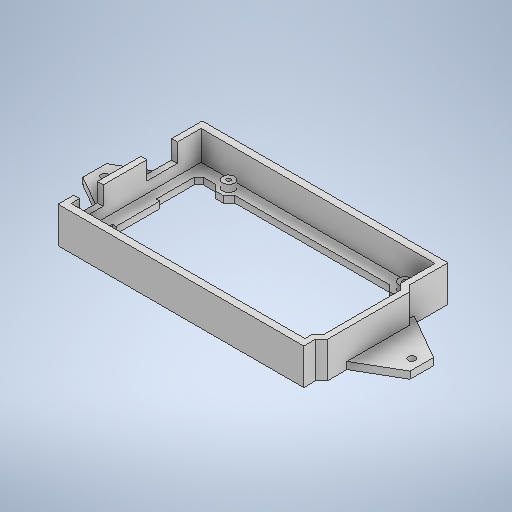
# Autodesk Inventor part: CaseArduinoMega
Saved by Autodesk Inventor 2025 (Build 290162000, 162)
## iProperties
Created: 2025-03-14
Part Number: CaseArduinoMega
Material: Genérico
Document SubType Name: Modeling
Designer: Ian
Density: 1 g/cm^3
Appearance: Padrão
Author: Ian
Autodesk Inventor part; units mm, degrees
ref_plane "YZ Plane" through (0, 0, 0) normal (1, 0, 0) x (0, 1, 0)
ref_plane "XZ Plane" through (0, 0, 0) normal (0, 1, 0) x (-1, 0, 0)
ref_plane "XY Plane" through (0, 0, 0) normal (0, 0, 1) x (1, 0, 0)
sketch "Esboço1" plane through (49, 0, -28.8005) normal (0, 1, 0) x (-1, 0, 0)
  line L0 (0, 16.5494) -> (0, 0)
  line L1 (0, 0) -> (0, 16.5494)
  line L2 (-2.54, 53.6742) -> (-2.54, 19.0894)
  line L3 (0, 16.5494) -> (-2.54, 19.0894)
  line L4 (-2.54, 19.0894) -> (-2.54, 53.6742)
  line L5 (-2.54, 53.6742) -> (0, 56.2142)
  line L6 (0, 56.2142) -> (0, 61.34)
  line L7 (104.54, 61.34) -> (104.54, 61.6011)
  line L8 (0, 61.34) -> (104.54, 61.34)
  line L9 (104.54, 61.34) -> (104.54, 0)
  line L10 (104.54, 0) -> (0, 0)
  line L11 (2.6222, 4.4772) -> (2.6222, 4.6028)
  line L12 (3.4259, 5.4351) -> (3.5514, 5.4395)
  circle A0 centre (11.8701, 6.54) radius 0.8973
  line L13 (8.9722, 52.7372) -> (8.9722, 52.8628)
  line L14 (9.7759, 53.6951) -> (9.9014, 53.6995)
  circle A1 centre (5.5202, 54.8) radius 0.8973
  line L15 (33.1022, 9.5572) -> (33.1022, 9.6828)
  line L16 (36.0001, 22.7395) -> (35.8746, 22.7351)
  circle A2 centre (35.9687, 21.84) radius 0.9
  line L17 (33.1022, 37.5628) -> (33.1022, 37.4372)
  line L18 (34.0314, 38.3995) -> (33.9059, 38.3951)
  circle A3 centre (36, 49.72) radius 0.8973
  line L19 (85.1722, 4.4772) -> (85.1722, 4.6028)
  line L20 (86.7372, 7.4351) -> (86.8627, 7.4395)
  circle A4 centre (86.8, 6.54) radius 0.9016
  circle A5 centre (88.07, 54.8) radius 0.8973
  dimension "d38" = 61.34
  dimension "d39" = 107.08
  dimension "d56" = 6.54
  dimension "d57" = 5.5202
  dimension "d58" = 6.54
  dimension "d60" = 21.84
  dimension "d61" = 38.5087
  dimension "d62" = 11.62
  dimension "d63" = 38.54
  dimension "d64" = 6.54
  dimension "d66" = 6.54
  dimension "d94" = 5.1258
  dimension "d95" = 16.5494
  dimension "d120" = 11.8701
  dimension "d121" = 16.47
  dimension "d122" = 17.74
  constraints: 42 end point, 4 centre point, 3 perpendicular, 2 collinear, 1 horizontal, 1 point on line, 1 vertical, 6 other
  measures "d38" distance between parallel lines of L10 L8
  measures "d39" distance between parallel lines of L9 L4
  measures "d56" distance from line of L8 A1.centre
  measures "d57" distance from line of L6 A1.centre
  measures "d58" distance from line of L10 A0.centre
  measures "d60" distance from line of L10 point (35.969, 21.84)
  measures "d61" distance from line of L2 point (35.969, 21.84)
  measures "d62" distance from line of L8 A3.centre
  measures "d63" distance from line of L2 A3.centre
  measures "d64" distance from line of L8 A5.centre
  measures "d66" distance from line of L10 point (86.8, 6.54)
  measures "d94" distance of L6.end L5.end
  measures "d95" distance of L0.end L0.start
  measures "d120" distance from line of L0 A0.centre
  measures "d121" distance from line of L9 A5.centre
  measures "d122" distance from line of L9 point (86.8, 6.54)
extrude "Extrusão1" add sketch "Esboço1" along normal blind 2.828
sketch "Esboço2" plane through (49, 2.828, -28.8005) normal (0, 1, 0) x (1, 0, 0)
  line L0 (-102.04, -58.34) -> (-102.04, -3)
  line L1 (0, 0) -> (-104.54, 0) projected
  line L2 (-104.54, -61.34) -> (0, -61.34) projected
  line L3 (-104.54, 0) -> (-104.54, -61.34) projected
  line L4 (-102.04, -3) -> (-2.5, -3)
  line L5 (-2.5, -58.34) -> (-102.04, -58.34)
  line L6 (-8.7044, -3) -> (1.4543, -3) construction
  line L7 (-2.5, -55.1787) -> (-2.5, -58.34)
  line L8 (2.54, -19.0894) -> (0, -16.5494) projected
  line L9 (2.54, -53.6742) -> (2.54, -19.0894) projected
  line L10 (0, -56.2142) -> (2.54, -53.6742) projected
  line L11 (0, -61.34) -> (0, -56.2142) projected
  line L12 (0, -16.5494) -> (0, 0) projected
  line L13 (0, 0) -> (0, -16.5494)
  line L14 (2.54, -19.0894) -> (2.54, -53.6742)
  line L15 (0, -56.2142) -> (0, -61.34)
  line L16 (-2.5, -55.1787) -> (0, -52.6787)
  line L17 (0, -20.0849) -> (-2.5, -17.5849)
  line L18 (-2.5, -17.5849) -> (-2.5, -3)
  line L19 (2.54, -19.0894) -> (0, -16.5494)
  line L20 (0, -20.0849) -> (0, -52.6787)
  point P0 (-49, -28.8005)
  point P1 (1.27, -54.9442)
  dimension "d3" = 3
  dimension "d4" = 3
  dimension "d6" = 2.5
  dimension "d15" = 2.5
  dimension "d96" = 2.5
  dimension "d97" = 2.5
  dimension "d98" = 2.5
  constraints: 26 end point, 4 parallel, 3 point on line, 2 collinear, 2 horizontal, 2 perpendicular, 2 vertical, 1 midpoint
  measures "d3" distance from line of L1 L0.end
  measures "d4" distance from line of L2 L0.start
  measures "d6" distance between parallel lines of L3 L0
  measures "d15" distance between parallel lines of L11 L7
  measures "d96" distance from line of point (1.27, -54.944) L16
  measures "d97" distance between parallel lines of L12 L18
  measures "d98" distance between parallel lines of L8 L17
extrude "Extrusão4" add sketch "Esboço2" along normal blind 12.5
sketch "Esboço5" plane through (-55.54, 0, -28.8005) normal (-1, 0, 0) x (0, 0, 1)
  line L0 (0, 0) -> (0, 15.328) projected
  line L1 (53.6742, 15.328) -> (19.0894, 15.328) projected
  line L2 (13.04, 15.328) -> (13.04, 7.478)
  line L3 (13.04, 7.478) -> (26.08, 7.478)
  line L4 (26.08, 7.478) -> (26.08, 15.328)
  line L5 (19.0894, 15.328) -> (26.08, 15.328)
  line L6 (55.1787, 15.328) -> (58.34, 15.328) projected
  line L7 (54.665, 15.328) -> (54.665, 7.478)
  line L8 (61.34, 0) -> (61.34, 15.328) projected
  line L9 (54.665, 7.478) -> (44.665, 7.478)
  line L10 (44.665, 7.478) -> (44.665, 15.328)
  line L11 (54.665, 15.328) -> (44.665, 15.328)
  line L12 (13.04, 15.328) -> (26.08, 15.328)
  line L13 (3, 15.328) -> (17.5849, 15.328) projected
  point P0 (28.8005, 0)
  point P1 (44.665, 11.403)
  point P2 (41.9718, 15.328)
  dimension "d45" = 13.04
  dimension "d46" = 13.04
  dimension "d47" = 7.85
  dimension "d49" = 7.85
  dimension "d50" = 6.675
  dimension "d51" = 10
  dimension "d52" = 18.585
  dimension "d53" = 61.34
  constraints: 18 end point, 4 point on line, 3 collinear, 3 perpendicular, 2 horizontal, 1 midpoint, 1 vertical
  measures "d45" distance between parallel lines of L0 L2
  measures "d46" distance of L2.end L3.end
  measures "d47" distance of L2.start L2.end
  measures "d49" distance of L7.start L7.end
  measures "d50" distance between parallel lines of L8 L7
  measures "d51" distance of L7.end L9.end
  measures "d52" distance from line of point (44.665, 11.403) L4
  measures "d53" distance between parallel lines of L8 L0
extrude "Extrusão5" cut sketch "Esboço5" against normal blind 12.5
sketch "Esboço7" plane through (-55.54, 0, -28.8005) normal (-1, 0, 0) x (0, 0, 1)
  line L0 (12.5489, 15.328) -> (31.9207, 15.328) projected
  line L1 (53.6742, 0) -> (19.0894, 0) projected
  line L2 (23.7839, 0) -> (33.7839, 0)
  line L3 (33.7839, 0) -> (33.7839, 3)
  line L4 (33.7839, 3) -> (23.7839, 3)
  line L5 (23.7839, 3) -> (23.7839, 0)
  point P0 (28.8005, 0)
  point P1 (39.5116, 15.328)
  point P2 (28.7839, 3)
  point P3 (28.7839, 0)
  point P4 (33.7839, 0)
  dimension "d68" = 10
  dimension "d69" = 3
  constraints: 8 end point, 2 midpoint, 2 parallel, 1 horizontal, 1 perpendicular, 1 point on line, 1 vertical alignment
  measures "d68" distance of L4.end L3.end
  measures "d69" distance of L3.end L2.end
extrude "Extrusão6" add sketch "Esboço7" along normal blind 17
sketch "Esboço10" plane through (51.54, 0, 24.8737) normal (1, 0, 0) x (0, 0, -1)
  line L0 (18.0042, 3) -> (28.0042, 3)
  line L1 (28.0042, 3) -> (28.0042, 0)
  line L2 (28.0042, 0) -> (18.0042, 0)
  line L3 (18.0042, 0) -> (18.0042, 3)
  line L4 (-7.6658, 15.328) -> (-2.54, 15.328) projected
  line L5 (-2.54, 15.328) -> (0, 15.328) projected
  line L6 (0, 15.328) -> (34.5848, 15.328) projected
  line L7 (34.5848, 15.328) -> (37.1248, 15.328) projected
  line L8 (37.1248, 15.328) -> (53.6742, 15.328) projected
  line L9 (-7.6658, 15.328) -> (53.6742, 15.328)
  line L10 (23.0042, 15.328) -> (23.0042, 6.8556)
  line L11 (-7.6658, 0) -> (-7.6658, 15.328) projected
  line L12 (0, 0) -> (34.5848, 0) projected
  point P0 (24.8737, 0)
  point P1 (23.0042, 3)
  dimension "d80" = 10
  dimension "d81" = 3
  dimension "d83" = 61.34
  dimension "d84" = 30.67
  dimension "d85" = 0
  dimension "d103" = 0
  constraints: 12 end point, 2 horizontal, 2 midpoint, 2 parallel, 2 perpendicular
  measures "d80" distance of L1.end L2.end
  measures "d81" distance of L0.end L1.end
  measures "d83" distance of L8.end L4.start
  measures "d84" distance between parallel lines of L11 L10
  measures "d85" distance from line of point (23.004, 3) L10
  measures "d103" distance between parallel lines of L12 L2
extrude "Extrusão9" add sketch "Esboço10" along normal blind 17
sketch "Esboço11" plane through (51.54, 3, 6.8695) normal (0, 1, 0) x (1, 0, 0)
  line L0 (17, 0) -> (17, 10) projected
  line L1 (-2.54, 19.1206) -> (-2.54, 35.67) projected
  line L2 (-2.54, 19.1206) -> (-2.54, 35.67) projected
  line L3 (0, 10) -> (17, 10) projected
  line L4 (17, 10) -> (-2.54, 21.2814)
  line L5 (0, -18.0042) -> (0, 16.5806) projected
  line L6 (17, 0) -> (0, -9.815)
  line L7 (0, 0) -> (17, 0) projected
  line L8 (0, 16.5806) -> (-2.54, 19.1206) projected
  line L9 (-2.54, 19.1206) -> (0, 16.5806)
  line L10 (-2.54, 21.2814) -> (-2.54, 19.1206)
  point P0 (-51.54, 6.8695)
  point P1 (-2.54, 21.2814)
  dimension "d99" = 30
  dimension "d100" = 30
  constraints: 8 end point, 2 collinear, 2 point on line
  measures "d99" angle of L3 L4
  measures "d100" angle of L6 L7
extrude "Extrusão11" add sketch "Esboço11" against normal up to surface (3 mm away) contours L6 L5 L7 | L3 L5 L8 L1 L4
sketch "Esboço12" plane through (-55.54, 3, 4.9834) normal (0, 1, 0) x (1, 0, 0)
  line L0 (0, 7.7039) -> (0, 20.7439) projected
  line L1 (-17, 10) -> (-17, 0) projected
  line L2 (-17, 0) -> (0, -9.815)
  line L3 (0, -20.8811) -> (0, -10.8811) projected
  line L4 (0, 10) -> (-17, 10) projected
  line L5 (-17, 10) -> (0, 19.815)
  line L6 (0, 0) -> (-17, 0) projected
  line L7 (0, 19.815) -> (0, 10)
  line L8 (0, 7.7039) -> (0, -10.8811) projected
  line L9 (-17, 10) -> (0, 10)
  line L10 (-17, 0) -> (0, 0)
  line L11 (0, -9.815) -> (0, 0)
  point P0 (55.54, 4.9834)
  dimension "d105" = 30
  dimension "d106" = 30
  constraints: 12 end point, 3 collinear, 2 point on line, 1 perpendicular
  measures "d105" angle of L4 L5
  measures "d106" angle of L6 L2
extrude "Extrusão12" add sketch "Esboço12" against normal up to surface (3 mm away) contours L4 L5 L0 | L8 L2 L6
sketch "Esboço13" plane through (-55.54, 3, 14.7983) normal (0, 1, 0) x (1, 0, 0)
  line L0 (0, -11.0661) -> (0, -1.0661) projected
  line L1 (-17, 9.815) -> (-17, 19.815) projected
  line L2 (0, 17.5189) -> (0, -1.0661) projected
  line L3 (0, 29.6299) -> (-17, 19.815) projected
  circle A0 centre (-12.75, 14.815) radius 1.5
  line L4 (124.08, 17.9289) -> (124.08, 7.9289) projected
  line L5 (107.08, -1.8861) -> (107.08, 24.5095) projected
  circle A1 centre (119.83, 12.9289) radius 1.5
  point P0 (55.54, 14.7983)
  dimension "d109" = 3
  dimension "d110" = 3
  constraints: 2 centre point
  measures "d109" diameter of A0
  measures "d110" diameter of A1
extrude "Extrusão13" cut sketch "Esboço13" against normal blind 10
sketch "Esboço14" plane through (49, 2.828, -28.8005) normal (0, 1, 0) x (1, 0, 0)
  circle A0 centre (-86.8, -6.54) radius 0.9016 projected
  circle A1 centre (-86.8, -6.54) radius 2.5
  circle A2 centre (-11.8701, -6.54) radius 0.8973 projected
  circle A3 centre (-11.8701, -6.54) radius 2.5
  circle A4 centre (-35.9687, -21.84) radius 0.9 projected
  circle A5 centre (-35.9687, -21.84) radius 2.5
  circle A6 centre (-88.07, -54.8) radius 0.8973 projected
  circle A7 centre (-88.07, -54.8) radius 2.5
  circle A8 centre (-36, -49.72) radius 0.8973 projected
  circle A9 centre (-36, -49.72) radius 2.5
  circle A10 centre (-5.5202, -54.8) radius 0.8973 projected
  circle A11 centre (-5.5202, -54.8) radius 2.5
  circle A12 centre (-36, -49.72) radius 0.8973 projected
  point P0 (-49, -28.8005)
  dimension "d113" = 5
  constraints: 6 centre point, 6 coincident, 3 equal radius
  measures "d113" diameter of A1
extrude "Extrusão14" add sketch "Esboço14" along normal blind 3
sketch "Esboço16" plane through (-39.07, 5.828, 25.9995) normal (0, 1, 0) x (1, 0, 0)
  line L0 (-13.97, 0.135) -> (-16.47, 0.135) projected
  line L1 (-16.47, 10.135) -> (-13.97, 10.135) projected
  line L2 (-13.97, 28.72) -> (-16.47, 28.72) projected
  line L3 (-16.47, 41.76) -> (-13.97, 41.76) projected
  line L4 (-9.97, 28.72) -> (-9.97, 44.8)
  line L5 (-8.47, 10.1069) -> (-8.47, 28.72)
  line L6 (85.57, -3.54) -> (-13.97, -3.54) projected
  line L7 (-13.97, 10.135) -> (-13.97, 0.135) projected
  line L8 (-7.9657, 46.8) -> (-2.8747, 46.8)
  line L9 (-0.3747, 44.3) -> (2.9148, 44.3)
  line L10 (5.4148, 46.8) -> (71.0558, 46.8)
  line L11 (88.07, 54.8) -> (-16.47, 54.8) projected
  line L12 (-16.47, -6.54) -> (88.07, -6.54) projected
  line L13 (90.61, 1.1258) -> (90.61, 35.7106) projected
  line L14 (-16.47, 28.72) -> (-16.47, 41.76) projected
  line L15 (-16.47, 28.72) -> (-16.47, 10.135) projected
  line L16 (-13.97, 51.8) -> (85.57, 51.8) projected
  circle A0 centre (1.2701, 48.26) radius 0.9016 projected
  circle A1 centre (0, 0) radius 0.8973 projected
  line L17 (-2.0287, 3.96) -> (2.0287, 3.96)
  line L18 (4.5287, 1.46) -> (77.3225, 1.46)
  line L19 (77.3225, 1.46) -> (78.4035, 1.46)
  line L20 (85.57, 51.8) -> (85.57, 37.2151) projected
  line L21 (85.57, 37.2151) -> (88.07, 34.7151) projected
  line L22 (88.07, 34.7151) -> (88.07, 2.1213) projected
  line L23 (80.07, 43.0238) -> (80.07, 35.7151)
  line L24 (80.07, 35.7151) -> (84.11, 31.3245)
  line L25 (84.11, 31.3245) -> (84.11, 6.8739)
  line L26 (80.07, 44.3) -> (80.07, 43.0238)
  line L27 (84.11, 3.96) -> (84.11, 6.8739)
  line L28 (73.5558, 44.3) -> (80.07, 44.3)
  circle A2 centre (76.2, 48.26) radius 0.8973 projected
  line L29 (73.7, 1.46) -> (77.7, 1.46) construction
  line L30 (78.4035, 1.46) -> (80.9035, 3.96)
  line L31 (78.4035, 1.46) -> (81.9391, 1.46) construction
  line L32 (80.9035, 3.96) -> (84.11, 3.96)
  line L33 (-16.47, 0.135) -> (-16.47, 10.135) projected
  line L34 (-9.97, 10.1069) -> (-8.47, 10.1069)
  line L35 (-9.97, 28.72) -> (-8.47, 28.72)
  line L36 (-7.9657, 46.8) -> (-7.97, 46.8)
  line L37 (-9.97, 44.8) -> (-7.97, 46.8)
  line L38 (-9.97, 44.8) -> (-7.1415, 44.8) construction
  line L39 (88.07, 38.2506) -> (88.07, 54.8) projected
  line L40 (71.0558, 46.8) -> (74.7636, 46.8) construction
  line L41 (71.0558, 46.8) -> (73.5558, 44.3)
  line L42 (71.0558, 46.8) -> (75.3342, 46.8) construction
  line L43 (-2.8747, 46.8) -> (-0.3747, 44.3)
  line L44 (2.9148, 44.3) -> (5.4148, 46.8)
  line L45 (-4.5287, 1.46) -> (-7.97, 1.46)
  line L46 (-4.5287, 1.46) -> (-2.0287, 3.96)
  line L47 (2.0287, 3.96) -> (4.5287, 1.46)
  line L48 (-9.97, 10.1069) -> (-9.97, 3.46)
  line L49 (-7.97, 1.46) -> (-9.97, 3.46)
  point P0 (39.07, 25.9995)
  point P1 (-9.97, 41.76)
  point P2 (1.2701, 44.3)
  point P3 (0, 3.96)
  point P4 (-15.22, 0.135)
  point P5 (-16.47, 35.24)
  point P6 (72.07, 46.8)
  point P7 (71.5558, 46.8)
  dimension "d131" = 8
  dimension "d157" = 6.5
  dimension "d158" = 8
  dimension "d162" = 2
  dimension "d165" = 8
  dimension "d166" = 6.5
  dimension "d167" = 8
  dimension "d170" = 2.5
  dimension "d172" = 2.5
  dimension "d173" = 2.5
  dimension "d174" = 2.5
  dimension "d175" = 2.5
  dimension "d176" = 2.5
  dimension "d177" = 2.5
  dimension "d180" = 8
  dimension "d181" = 2.5
  dimension "d182" = 2.5
  dimension "d183" = 2.5
  dimension "d184" = 2
  dimension "d185" = 2
  dimension "d186" = 2
  constraints: 66 end point, 11 horizontal, 6 parallel, 6 point on line, 4 midpoint, 4 perpendicular, 2 collinear, 2 equal length, 2 vertical, 2 vertical alignment
  measures "d131" distance between parallel lines of L11 L10
  measures "d157" distance from line of L4 point (-16.47, 35.24)
  measures "d158" distance between parallel lines of L15 L5
  measures "d162" horizontal distance of L4.end L36.end
  measures "d165" distance between parallel lines of L12 L18
  measures "d166" distance between parallel lines of L13 L25
  measures "d167" distance between parallel lines of L39 L23
  measures "d170" distance between parallel lines of L10 L28
  measures "d172" distance between parallel lines of L9 L8
  measures "d173" horizontal distance of L8.end L9.start
  measures "d174" horizontal distance of L9.end L10.start
  measures "d175" distance between parallel lines of L18 L17
  measures "d176" horizontal distance of L45.start L17.start
  measures "d177" horizontal distance of L17.end L18.start
  measures "d180" distance from line of point (72.07, 46.8) L23
  measures "d181" horizontal distance of L19.end L30.end
  measures "d182" distance between parallel lines of L32 L19
  measures "d183" horizontal distance of L10.end L28.start
  measures "d184" horizontal distance of L4.end L36.end
  measures "d185" horizontal distance of L45.end L48.end
  measures "d186" horizontal distance of L45.end L48.end
extrude "Extrusão15" cut sketch "Esboço16" against normal blind 10 contours L4 L37 L36 L8 L43 L9 L44 L10 L41 L28 L26 L23 L24 L25 L27 L32 L30 L19 L18 L47 L17 L46 L45 L49 L48 L34 L5 L35
equation "\"d84\" = 0.5 * d83"
